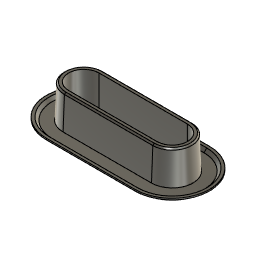
SPILLWAYliner (Autodesk Fusion 360 design; units mm, degrees)
Autodesk Fusion 360 part; units mm, degrees
sketch "Sketch1" plane through (0, 0, 0) normal (0, 0, 1) x (1, 0, 0)
  line L0 (23.5, 7.5) -> (-23.5, 7.5)
  line L1 (-23.5, 7.5) -> (-23.5, -7.5)
  line L2 (-23.5, -7.5) -> (23.5, -7.5)
  line L3 (23.5, -7.5) -> (23.5, 7.5)
  line L4 (23.5, 7.5) -> (-23.5, -7.5) construction
  line L5 (-23.5, 7.5) -> (23.5, -7.5) construction
  dimension "d1" = 47
  dimension "d2" = 15
  constraint horizontal L0
  constraint perpendicular L0 L1
  constraint parallel L0 L2
  constraint parallel L1 L3
  constraint coincident L4 origin
  constraint coincident L5 origin
  measures "d1" distance of L1.end L2.end
  measures "d2" distance of L0.end L1.end
extrude "Extrude1" add sketch "Sketch1" along normal blind 2 thin wall 6 outside
extrude "Extrude3" add sketch "Sketch1" along normal blind 13 thin wall 2 inside
extrude "Extrude4" cut sketch "Sketch1" along normal blind 1 from surface at 1 thin wall 4 outside
fillet "Fillet1" radius 5.5 4 edges at (21.5, 5.5, 6.5) (21.5, -5.5, 6.5) (-21.5, 5.5, 6.5) (-21.5, -5.5, 6.5)
fillet "Fillet1" radius 7.5 4 edges at (-23.5, 7.5, 7) (23.5, -7.5, 7) (-23.5, -7.5, 7) (23.5, 7.5, 7)
fillet "Fillet1" radius 11.5 4 edges at (-27.5, 11.5, 1.5) (27.5, 11.5, 1.5) (-27.5, -11.5, 1.5) (27.5, -11.5, 1.5)
fillet "Fillet1" radius 13.5 4 edges at (29.5, -13.5, 1) (29.5, 13.5, 1) (-29.5, -13.5, 1) (-29.5, 13.5, 1)
chamfer "Chamfer1" distance 1 angle 45 4 edges at (-27.5, 0, 2) (0, -11.5, 2) (27.5, 0, 2) (0, 11.5, 2)
chamfer "Chamfer1" distance 1.5 angle 45 4 edges at (0, -5.5, 0) (21.5, 0, 0) (0, 5.5, 0) (-21.5, 0, 0)
chamfer "Chamfer1" distance 12 distance2 0.5 4 edges at (23.5, 0, 13) (0, -7.5, 13) (-23.5, 0, 13) (0, 7.5, 13) measured on face at (23.5, -0.0005, 5) measured on face at (5.3337, -6.8333, 13) measured on face at (-23.5, 0.0005, 5) measured on face at (5.3337, -6.8333, 13)
chamfer "Chamfer1" distance 1.5 distance2 2 4 edges at (29.5, 0, 0) (0, 13.5, 0) (-29.5, 0, 0) (0, -13.5, 0) measured on face at (29.5, -0.0009, 0.6667) measured on face at (5.3342, 13.5, 0.6667) measured on face at (-29.5, 0.0009, 0.6667) measured on face at (-5.3342, -13.5, 0.6667)
chamfer "Chamfer2" distance 0.5 angle 45 4 edges at (23, 0, 13) (0, -7, 13) (-23, 0, 13) (0, 7, 13)
component "body" placed x (1, 0, 0) y (0, 1, 0) z (0, 0, 1) at (0, 0, 0)
